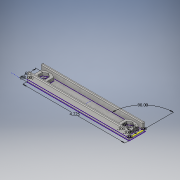
# Autodesk Inventor part: LiDAR_mount_sweepclamp_Rev.1
Saved by Autodesk Inventor 2016 (Build 200138000, 138)
## iProperties
Created: 2018-03-02
Part Number: LiDAR_mount_sweepclamp_Rev.1
Material: Generic
Document SubType Name: Modeling
Designer: emvanzant
Density: 1 g/cm^3
Appearance: Default
Sheet Metal Rule: Default
Author: emvanzant
Autodesk Inventor part; units mm, degrees
ref_plane "YZ Plane" through (0, 0, 0) normal (1, 0, 0) x (0, 1, 0)
ref_plane "XZ Plane" through (0, 0, 0) normal (0, 1, 0) x (-1, 0, 0)
ref_plane "XY Plane" through (0, 0, 0) normal (0, 0, 1) x (1, 0, 0)
sketch "Sketch1" plane through (0, 0, 0) normal (0, 1, 0) x (-1, 0, 0)
  line L0 (0, 0) -> (107.315, 0)
  line L1 (107.315, 0) -> (107.315, -17.145)
  line L2 (107.315, 0) -> (124.46, 0) construction
  line L3 (107.315, -17.145) -> (0, -17.145)
  line L4 (0, -17.145) -> (0, 0)
  dimension "d0" = 107.315
  dimension "d1" = 17.145
  dimension "d2" = 90
  constraints: 10 end point, 3 perpendicular, 2 horizontal, 1 vertical
  measures "d0" distance of L0.start L0.end
  measures "d1" distance of L0.end L1.end
  measures "d2" angle of L1 L2
extrude "Extrusion1" add sketch "Sketch1" along normal blind 2.54
sketch "Sketch2" plane through (0, 2.54, 0) normal (0, 1, 0) x (1, 0, 0)
  line L0 (0, 0) -> (0, 17.145) projected
  line L1 (0, 8.5725) -> (-9.2075, 8.5725) construction
  line L2 (0, 8.5725) -> (-2.576, 8.5725)
  line L3 (-2.576, 8.5725) -> (-2.576, 12.4012)
  line L4 (-2.576, 8.5725) -> (-2.576, 4.7438)
  line L5 (0, 17.145) -> (0, 14.605)
  line L6 (0, 14.605) -> (-107.315, 14.605)
  line L7 (-107.315, 17.145) -> (-107.315, 0) projected
  line L8 (-107.315, 14.605) -> (-107.315, 17.145)
  line L9 (0, 17.145) -> (-107.315, 17.145) projected
  line L10 (-107.315, 17.145) -> (0, 17.145)
  line L11 (0, 0) -> (0, 2.54)
  line L12 (0, 2.54) -> (-107.315, 2.54)
  line L13 (-107.315, 0) -> (0, 0)
  line L14 (-2.576, 12.4012) -> (-6.3932, 14.605)
  line L15 (-6.3932, 14.605) -> (-12.032, 14.605)
  line L16 (-2.576, 4.7438) -> (-6.3932, 2.54)
  line L17 (-12.032, 14.605) -> (-15.839, 12.4071)
  line L18 (-15.839, 12.4071) -> (-15.839, 4.7438)
  line L19 (-15.839, 4.7438) -> (-12.0218, 2.54)
  line L20 (-9.2075, 13.2969) -> (-5.116, 10.9347)
  line L21 (-5.116, 10.9347) -> (-5.116, 6.2103)
  line L22 (-5.116, 6.2103) -> (-9.2075, 3.8481)
  line L23 (-9.2075, 3.8481) -> (-13.299, 6.2103)
  line L24 (-13.299, 6.2103) -> (-13.299, 10.9347)
  line L25 (-13.299, 10.9347) -> (-9.2075, 13.2969)
  line L26 (-53.6575, 14.605) -> (-53.6575, 2.54) construction
  line L27 (-107.315, 8.5725) -> (-98.1075, 8.5725) construction
  line L28 (-107.315, 8.5725) -> (-104.739, 8.5725)
  line L29 (-104.739, 8.5725) -> (-104.739, 12.4012)
  line L30 (-104.739, 8.5725) -> (-104.739, 4.7438)
  line L31 (-104.739, 12.4012) -> (-100.9218, 14.605)
  line L32 (-104.739, 4.7438) -> (-100.9218, 2.54)
  line L33 (-95.283, 14.605) -> (-91.476, 12.4071)
  line L34 (-91.476, 12.4071) -> (-91.476, 4.7438)
  line L35 (-91.476, 4.7438) -> (-95.2932, 2.54)
  line L36 (-98.1075, 8.5725) -> (-98.1075, 14.605)
  line L37 (-98.1075, 13.2969) -> (-102.199, 10.9347)
  line L38 (-102.199, 10.9347) -> (-102.199, 6.2103)
  line L39 (-102.199, 6.2103) -> (-98.1075, 3.8481)
  line L40 (-98.1075, 3.8481) -> (-94.016, 6.2103)
  line L41 (-94.016, 6.2103) -> (-94.016, 10.9347)
  line L42 (-94.016, 10.9347) -> (-98.1075, 13.2969)
  line L43 (-100.9218, 14.605) -> (-95.283, 14.605)
  line L44 (-100.9218, 2.54) -> (-95.2932, 2.54)
  point P0 (-8.3776, 2.54)
  point P1 (-9.2075, 14.605)
  dimension "d5" = 9.2075
  dimension "d16" = 2.54
  dimension "d17" = 90
  dimension "d18" = 2.54
  dimension "d20" = 5.6388
  dimension "d30" = 4.7244
  dimension "d43" = 2.54
  dimension "d44" = 2.54
  dimension "d45" = 2.54
  dimension "d46" = 2.54
  constraints: 84 end point, 20 symmetric about line, 13 point on line, 4 parallel, 3 midpoint, 2 coincident, 2 collinear, 2 vertical, 1 horizontal, 1 perpendicular, 13 other
  measures "d5" distance of L1.start L1.end
  measures "d16" distance of L0.end L5.end
  measures "d17" angle of L5 L6
  measures "d18" distance of L0.start L11.end
  measures "d20" distance of L14.end L15.end
  measures "d30" distance of L20.start L20.end
  measures "d43" distance between parallel lines of L16 L22
  measures "d44" distance between parallel lines of L3 L21
  measures "d45" distance between parallel lines of L18 L24
  measures "d46" distance between parallel lines of L19 L23
hole "Hole1" at (-9.2075, 2.54, -8.5725) direction (0, -1, 0) diameter 3.81 end through all
extrude "Extrusion2" add sketch "Sketch2" along normal blind 6.35 contours L13 L7 L12 L0 | L6 L7 L9 L0
extrude "Extrusion4" add sketch "Sketch2" along normal blind 3.175 contours L12 L19 L18 L17 L6 L14 L3 L4 L16 | L32 L30 L29 L31 L6 L33 L34 L35 L12
hole "Hole2" at (-98.1075, 2.54, -8.5725) direction (0, -1, 0) diameter 3.81 end through all
fillet "Fillet1" radius 0.7874 22 edges at (-107.315, 0, -8.5725) (-53.6575, 0, 0) (-53.6575, 0, -17.145) (0, 0, -8.5725) (-107.315, 4.445, -17.145) (-107.315, 5.715, -14.605) (-107.315, 2.54, -8.5725) (-107.315, 5.715, -2.54) (-107.315, 4.445, 0) (-107.315, 8.89, -1.27) (-107.315, 8.89, -15.875) (-53.6575, 8.89, -17.145) (-53.6575, 8.89, -14.605) (-53.6575, 8.89, -2.54) (-53.6575, 8.89, 0) (0, 8.89, -1.27) (0, 4.445, 0) (0, 5.715, -2.54) (0, 2.54, -8.5725) (0, 5.715, -14.605) (0, 4.445, -17.145) (0, 8.89, -15.875)
equation "\"BendRadius\" = Thickness"
equation "\"BendReliefWidth\" = Thickness"
equation "\"BendReliefDepth\" = 0.5 * Thickness"
equation "\"CornerReliefSize\" = 4 * Thickness"
equation "\"MinimumRemnant\" = 2 * Thickness"
equation "\"TransitionRadius\" = BendRadius"
equation "\"JacobiRadiusSize\" = Thickness"
equation "\"GapSize\" = Thickness"
equation "\"Thickness\" = 3.048"
body "Solid1"
